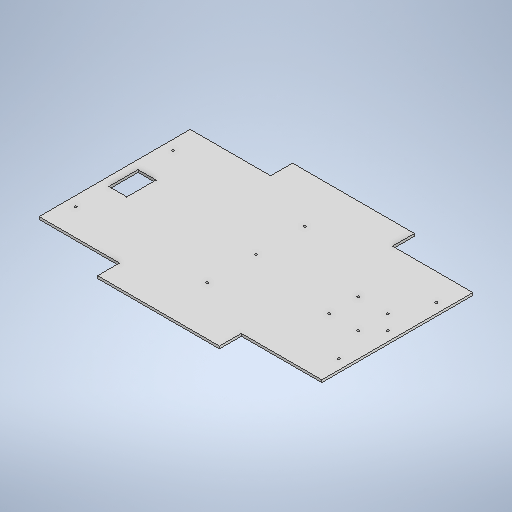
# Autodesk Inventor part: вверхняя плита
Saved by Autodesk Inventor 2025 (Build 290162000, 162)
## iProperties
Created: 2025-02-24
Part Number: вверхняя плита
Material: Типовые
Document SubType Name: Modeling
Designer: volko
Density: 1 g/cm^3
Appearance: По умолчанию
Author: volko
Autodesk Inventor part; units mm, degrees
ref_plane "YZ Plane" through (0, 0, 0) normal (1, 0, 0) x (0, 1, 0)
ref_plane "XZ Plane" through (0, 0, 0) normal (0, 1, 0) x (-1, 0, 0)
ref_plane "XY Plane" through (0, 0, 0) normal (0, 0, 1) x (1, 0, 0)
sketch "Эскиз1" plane through (0, 0, 0) normal (0, 1, 0) x (-1, 0, 0)
  line L0 (-290, 155) -> (-290, -155)
  line L1 (290, -155) -> (290, 155)
  line L2 (0, -280) -> (0, 280) projected
  line L3 (406, 0) -> (-406, 0) projected
  line L4 (125, 155) -> (125, 200)
  line L5 (125, 200) -> (-125, 200)
  line L6 (-125, 200) -> (-125, 155)
  line L7 (290, 155) -> (125, 155)
  line L8 (-125, 155) -> (-290, 155)
  line L9 (125, -155) -> (125, -200)
  line L10 (125, -200) -> (-125, -200)
  line L11 (-125, -200) -> (-125, -155)
  line L12 (-290, -155) -> (-125, -155)
  line L13 (125, -155) -> (290, -155)
  line L14 (272, -30) -> (235, -30)
  line L15 (235, -30) -> (235, 30)
  line L16 (235, 30) -> (272, 30)
  line L17 (272, 30) -> (272, -30)
  point P0 (0, 0)
  dimension "d0" = 580
  dimension "d1" = 310
  dimension "d39" = 400
  dimension "d40" = 250
  dimension "d41" = 18
  dimension "d42" = 60
  dimension "d43" = 55
  constraints: 32 end point, 7 parallel, 5 perpendicular, 4 symmetric about line, 3 horizontal, 1 collinear, 1 vertical, 5 other
  measures "d0" distance of L1.end L0.start
  measures "d1" distance of L1.start L1.end
  measures "d39" distance between parallel lines of L10 L5
  measures "d40" distance of L4.end L5.end
  measures "d41" distance between parallel lines of L17 L1
  measures "d42" distance between parallel lines of L16 L14
  measures "d43" distance between parallel lines of L15 L1
extrude "Выдавливание1" add sketch "Эскиз1" along normal blind 5 contours L8 L6 L5 L2 L3 L0 | L3 L2 L10 L11 L12 L0 | L3 L15 L14 L17 L1 L13 L9 L10 L2 | L2 L5 L4 L7 L1 L3 L17 L16 L15
sketch "Эскиз2" plane through (0, 5, 0) normal (0, 1, 0) x (1, 0, 0)
  line L0 (0, 280) -> (0, -280) projected
  line L1 (-406, 0) -> (406, 0) projected
  point P0 (0, 0)
  point P1 (240, 30)
  point P2 (0, 0)
  point P3 (270, 100)
  point P4 (180, 30)
  point P5 (240, -30)
  point P6 (180, -30)
  point P7 (0, 100)
  point P8 (270, 0)
  point P9 (0, 0)
  point P10 (270, -100)
  point P11 (0, -100)
  point P12 (-270, 100)
  point P13 (-270, -100)
  dimension "d15" = 60
  dimension "d18" = 60
  dimension "d21" = 180
  dimension "d22" = 270
  dimension "d32" = 270
  dimension "d35" = 100
  constraints: 4 symmetric about line, 2 horizontal, 2 vertical, 1 coincident, 8 other
  measures "d15" distance of point (240, 30) point (180, 30)
  measures "d18" distance of point (240, 30) point (240, -30)
  measures "d21" distance from line of L0 point (180, 30)
  measures "d22" distance from line of point (270, 100) L0
  measures "d32" distance of point (270, 100) point (0, 100)
  measures "d35" distance of point (270, 100) point (270, 0)
hole "Отверстие1" at (0, 5, -100) at (0, 5, 100) at (0, 5, 0) at (180, 5, 30) at (180, 5, -30) at (240, 5, 30) at (240, 5, -30) at (270, 5, 100) at (270, 5, 0) at (270, 5, -100) at (-270, 5, 100) at (-270, 5, -100) direction (0, -1, 0) diameter 4.5 end through all
